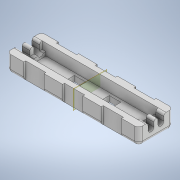
# Autodesk Inventor part: DupontSkarv
Saved by Autodesk Inventor 2021 (Build 250183000, 183)
## iProperties
Created: 2025-01-16
Part Number: DupontSkarv
Material: Generic
Document SubType Name: Modeling
Designer: 24oscnor
Density: 1 g/cm^3
Appearance: Default
Author: 24oscnor
Autodesk Inventor part; units mm, degrees
ref_plane "YZ Plane" through (0, 0, 0) normal (1, 0, 0) x (0, 1, 0)
ref_plane "XZ Plane" through (0, 0, 0) normal (0, 1, 0) x (-1, 0, 0)
ref_plane "XY Plane" through (0, 0, 0) normal (0, 0, 1) x (1, 0, 0)
sketch "Sketch1" plane through (0, 0, 0) normal (0, 1, 0) x (-1, 0, 0)
  line L0 (0, 0) -> (15, 0)
  line L1 (15, 0) -> (15, 5.28)
  line L2 (15, 5.28) -> (0, 5.28)
  line L3 (0, 5.28) -> (0, 0)
  line L4 (12, 0.64) -> (9, 0.64)
  line L5 (9, 0.64) -> (9, 4.64)
  line L6 (9, 4.64) -> (12, 4.64)
  line L7 (12, 4.64) -> (12, 0.64)
  dimension "d0" = 15
  dimension "d1" = 5.28
  dimension "d17" = 3
  dimension "d18" = 0.64
  dimension "d19" = 0.64
  dimension "d20" = 3
  constraints: 16 end point, 4 parallel, 2 horizontal, 2 perpendicular
  measures "d0" distance of L1.end L2.end
  measures "d1" distance of L2.end L0.start
  measures "d17" distance between parallel lines of L5 L7
  measures "d18" distance between parallel lines of L2 L6
  measures "d19" distance between parallel lines of L4 L0
  measures "d20" distance between parallel lines of L1 L7
extrude "Extrusion1" add sketch "Sketch1" along normal blind 1.46
sketch "Sketch2" plane through (0, 0, 5.28) normal (1, 0, 0) x (0, 0, -1)
  circle A0 centre (1.37, 2.73) radius 0.75
  line L0 (0, 1.46) -> (5.28, 1.46) projected
  line L1 (0, 0) -> (0, 1.46) projected
  line L2 (5.28, 0) -> (0, 0) projected
  line L3 (2.64, 0) -> (2.64, 4.8627)
  line L4 (0.62, 2.73) -> (0.62, 3.763)
  circle A1 centre (0, 3.763) radius 0.62
  line L5 (2.12, 2.73) -> (2.12, 3.763)
  circle A2 centre (2.64, 3.763) radius 0.52
  circle A3 centre (3.91, 2.73) radius 0.75
  line L6 (4.66, 2.73) -> (4.66, 3.763)
  circle A4 centre (5.28, 3.763) radius 0.62
  line L7 (3.16, 2.73) -> (3.16, 3.763)
  circle A5 centre (2.64, 3.763) radius 0.52
  line L8 (0, 0) -> (0, 1.46) projected
  line L9 (5.28, 1.46) -> (0, 1.46) projected
  line L10 (5.28, 1.46) -> (5.28, 3.763)
  line L11 (0, 3.763) -> (0, 1.46)
  line L12 (0, 3.763) -> (0, 4.383)
  line L13 (5.28, 3.763) -> (5.28, 4.383)
  line L14 (0, 1.46) -> (5.28, 1.46)
  line L15 (5.28, 1.46) -> (5.28, 0)
  line L16 (5.28, 0) -> (0, 0)
  line L17 (0, 0) -> (0, 1.46)
  dimension "d13" = 1.04
  dimension "d4" = 1.27
  dimension "d5" = 1.5
  dimension "d6" = 1.37
  dimension "d7" = 1.033
  dimension "d9" = 1.24
  dimension "d10" = 2.303
  dimension "d11" = 1.033
  dimension "d12" = 0.75
  constraints: 26 end point, 8 point on circle, 6 symmetric about line, 5 vertical, 4 centre point, 3 parallel, 1 horizontal, 1 horizontal alignment, 1 midpoint, 1 perpendicular, 1 point on line, 1 tangent, 7 other
  measures "d4" distance from line of L0 A0.centre
  measures "d5" diameter of A0
  measures "d6" distance from line of A0.centre L1
  measures "d7" distance of L4.start L4.end
  measures "d9" diameter of A1
  measures "d10" distance from line of L0 L11.start
  measures "d11" distance of L5.start L5.end
  measures "d12" distance from line of A0.centre L5
extrude "Extrusion2" add sketch "Sketch2" along normal blind 2 contours L5 A2 L3 L0 L11 A1 L4 A0 | A2 L3 | A1 L11 L12 | A2 L3 | A2 L7 A3 L6 A4 L10 L0 L3 | L3 L2 L1 L0 | L0 L15 L2 L3 | A4 L13 L10 picked at (0.2185, 4.1108) picked at (4.8923, 3.8987)
sketch "Sketch3" plane through (0, 0, 0) normal (0, 1, 0) x (-1, 0, 0)
  line L0 (-2, 5.28) -> (-2, 0) projected
  line L1 (-2, 0) -> (15, 0)
  line L2 (15, 0) -> (15, -1.32)
  line L3 (15, -1.32) -> (-2, -1.32)
  line L4 (-2, -1.32) -> (-2, 0)
  line L5 (15, 0) -> (15, 5.28) projected
  line L6 (-2, -1.32) -> (2.4, -1.32)
  line L7 (2.4, -1.32) -> (2.4, -1.82)
  line L8 (2.4, -1.82) -> (-2, -1.82)
  line L9 (-2, -1.82) -> (-2, -1.32)
  line L10 (7.6, -1.32) -> (12.4, -1.32)
  line L11 (12.4, -1.32) -> (12.4, -1.82)
  line L12 (12.4, -1.82) -> (7.6, -1.82)
  line L13 (7.6, -1.82) -> (7.6, -1.32)
  line L14 (-2, 2.64) -> (25.5068, 2.64)
  line L15 (-2, 0) -> (-2, 5.28)
  line L16 (-2, 5.28) -> (15, 5.28)
  line L17 (15, 5.28) -> (15, 6.6)
  line L18 (15, 6.6) -> (-2, 6.6)
  line L19 (-2, 6.6) -> (-2, 5.28)
  line L20 (15, 5.28) -> (15, 0)
  line L21 (-2, 6.6) -> (2.4, 6.6)
  line L22 (2.4, 6.6) -> (2.4, 7.1)
  line L23 (2.4, 7.1) -> (-2, 7.1)
  line L24 (-2, 7.1) -> (-2, 6.6)
  line L25 (7.6, 6.6) -> (12.4, 6.6)
  line L26 (12.4, 6.6) -> (12.4, 7.1)
  line L27 (12.4, 7.1) -> (7.6, 7.1)
  line L28 (7.6, 7.1) -> (7.6, 6.6)
  point P0 (0, 0)
  point P1 (0, 5.28)
  point P2 (2.4, -1.32)
  dimension "d21" = 1.32
  dimension "d22" = 0
  dimension "d23" = 4.4
  dimension "d24" = 0.5
  dimension "d25" = 0.5
  dimension "d26" = 5.2
  dimension "d27" = 2.6
  constraints: 54 end point, 15 symmetric about line, 6 parallel, 4 horizontal, 3 perpendicular, 2 point on line, 1 midpoint
  measures "d21" distance between parallel lines of L1 L3
  measures "d22" distance between parallel lines of L5 L2
  measures "d23" distance between parallel lines of L9 L7
  measures "d24" distance between parallel lines of L3 L8
  measures "d25" distance between parallel lines of L3 L12
  measures "d26" distance between parallel lines of L13 L7
  measures "d27" distance between parallel lines of L2 L11
extrude "Extrusion3" add sketch "Sketch3" along normal blind 4.383 contours L19 L18 L17 L16 | L24 L23 L22 L18 | L1 L2 L3 L4 | L3 L7 L8 L9 | L18 L28 L27 L26 | L11 L12 L13 L3
fillet "Fillet1" radius 1 5 edges at (2, 2.1915, -1.82) (2, 0, 2.64) (-0.2, 0, -1.82) (2, 2.1915, 7.1) (-0.2, 0, 7.1)
sketch "Sketch4" plane through (0, 0, 5.28) normal (-1, 0, 0) x (0, 0, 1)
  arc A0 (-4.66, 2.73) -> (-3.16, 2.73) centre (-3.91, 2.73) ccw projected
  circle A1 centre (-3.91, 2.73) radius 0.75
  line L0 (-4.6097, 2.46) -> (-5.28, 2.46)
  line L1 (-5.28, 1.46) -> (-5.28, 4.383) projected
  line L2 (-5.28, 1.46) -> (0, 1.46) projected
  line L3 (-5.28, 2.46) -> (-5.28, 1.46)
  line L4 (-5.28, 1.46) -> (0, 1.46)
  arc A2 (-2.12, 3.763) -> (-3.16, 3.763) centre (-2.64, 3.763) ccw projected
  line L5 (-2.64, 4.283) -> (-2.64, 1.46)
  line L6 (-4.64, 1.46) -> (-0.64, 1.46) projected
  arc A3 (-2.12, 2.73) -> (-0.62, 2.73) centre (-1.37, 2.73) ccw
  circle A4 centre (-1.37, 2.73) radius 0.75
  line L7 (-0.6703, 2.46) -> (0, 2.46)
  line L8 (0, 1.46) -> (0, 4.383)
  line L9 (0, 1.46) -> (-5.28, 1.46)
  line L10 (0, 2.46) -> (0, 1.46)
  line L11 (0, 1.46) -> (-5.28, 1.46)
  line L12 (-0.64, 1.46) -> (-4.64, 1.46)
  line L13 (-3.2103, 2.46) -> (-2.64, 2.46)
  line L14 (-2.0697, 2.46) -> (-2.64, 2.46)
  point P0 (-5.28, 0)
  dimension "d31" = 1
  dimension "d32" = 90
  dimension "d33" = 0.5703
  constraints: 24 end point, 12 symmetric about line, 8 point on circle, 3 centre point, 3 point on line, 2 coincident, 1 collinear, 1 horizontal, 1 midpoint, 1 perpendicular, 1 vertical, 2 other
  measures "d31" distance between parallel lines of L0 L2
  measures "d32" angle of L5 L2
  measures "d33" distance of L13.start L13.end
extrude "Extrusion4" add sketch "Sketch4" along normal blind 1 contours A0 L13 L5 L2 L1 L0 | L14 A3 L7 L8 L2 L5
ref_plane "Work Plane1" through (-15, 1.46, 5.28) normal (-1, 0, 0) x (0, 0, 1)
mirror "Mirror1" about plane through (-15, 1.46, 5.28) normal (-1, 0, 0) of "Extrusion3", "Extrusion2", "Extrusion4", "Extrusion1", "Fillet1"
body "Solid1"
